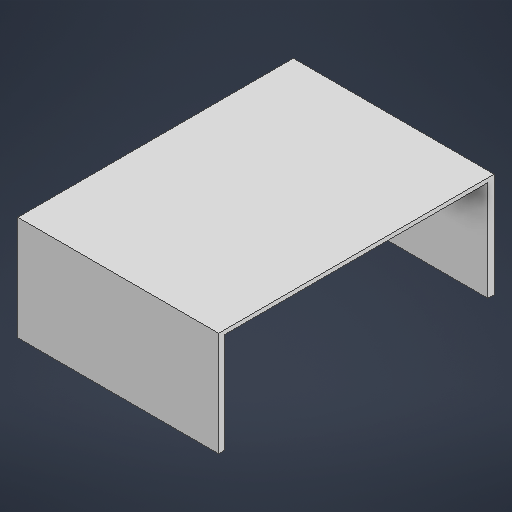
# Autodesk Inventor part: Module Cover
Saved by Autodesk Inventor 2027 (Build 310192060, 192F)
## iProperties
Created: 2026-06-22
Part Number: Module Cover
Material: Generic
Document SubType Name: Modeling
Designer: cfang
Density: 1 g/cm^3
Appearance: Default
Author: cfang
Autodesk Inventor part; units mm, degrees
ref_plane "YZ Plane" through (0, 0, 0) normal (1, 0, 0) x (0, 1, 0)
ref_plane "XZ Plane" through (0, 0, 0) normal (0, 1, 0) x (-1, 0, 0)
ref_plane "XY Plane" through (0, 0, 0) normal (0, 0, 1) x (1, 0, 0)
sketch "Sketch1" plane through (0, 0, 0) normal (0, 1, 0) x (-1, 0, 0)
  line L0 (-24.05, -31.5) -> (24.05, -31.5)
  line L1 (24.05, -31.5) -> (24.05, 31.5)
  line L2 (24.05, 31.5) -> (-24.05, 31.5)
  line L3 (-24.05, 31.5) -> (-24.05, -31.5)
  line L4 (-24.05, -31.5) -> (24.05, 31.5) construction
  line L5 (24.05, -31.5) -> (-24.05, 31.5) construction
  point P0 (0, 0)
  dimension "d0" = 63
  dimension "d1" = 48.1
  constraints: 12 end point, 2 midpoint, 2 parallel, 1 horizontal, 1 perpendicular
  measures "d0" distance of L0.end L1.end
  measures "d1" distance of L1.end L2.end
extrude "Extrusion1" add sketch "Sketch1" along normal blind 1
sketch "Sketch2" plane through (0, 1, 0) normal (0, 1, 0) x (1, 0, 0)
  line L0 (-24.05, -31.5) -> (24.05, -31.5) projected
  line L1 (-24.05, -31.5) -> (24.05, -31.5)
  line L2 (24.05, -31.5) -> (24.05, -33)
  line L3 (24.05, -33) -> (-24.05, -33)
  line L4 (-24.05, -33) -> (-24.05, -31.5)
  line L5 (-24.05, 31.5) -> (24.05, 31.5)
  line L6 (24.05, 31.5) -> (24.05, 33)
  line L7 (24.05, 33) -> (-24.05, 33)
  line L8 (-24.05, 33) -> (-24.05, 31.5)
  point P0 (0, 0)
  point P1 (20.95, -31.5)
  dimension "d4" = 1.5
  constraints: 16 end point, 4 parallel, 2 horizontal, 2 perpendicular, 2 point on line, 1 coincident, 1 collinear
  measures "d4" distance of L3.end L0.start
extrude "Extrusion2" add sketch "Sketch2" against normal blind 25
body "Solid1"
